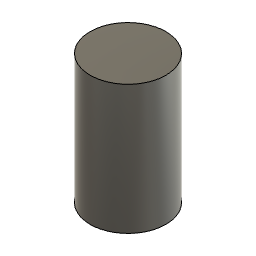
Busylight v2 (Autodesk Fusion 360 design; units mm, degrees)
Autodesk Fusion 360 part; units mm, degrees
sketch "Esquisse1" plane through (0, 0, 0) normal (0, 1, 0) x (1, 0, 0)
  circle A0 centre (0, 0) radius 12.5
  line L0 (12.5, 0) -> (0.5, 0) construction
  line L1 (-12.5, 0) -> (-4.5, 0) construction
  line L2 (-4.5, 6.25) -> (0.5, 6.25)
  line L3 (0.5, 6.25) -> (0.5, -6.25)
  line L4 (0.5, -6.25) -> (-4.5, -6.25)
  line L5 (-4.5, -6.25) -> (-4.5, 6.25)
  dimension "d1" = 25
  dimension "d2" = 12
  dimension "d3" = 8
  dimension "d4" = 12.5
  constraint coincident A0.centre origin
  constraint coincident A0 L0.start
  constraint horizontal L0
  constraint horizontal L1
  constraint coincident A0 L1.start
  constraint horizontal L2
  constraint vertical L3
  constraint horizontal L4
  constraint vertical L5
  constraint midpoint L0.end L3
  measures "d1" diameter of A0
  measures "d2" distance of L0.start L0.end
  measures "d3" distance of L1.start L1.end
  measures "d4" distance of L2.start L4.end
extrude "Extrusion1" add sketch "Esquisse1" along normal blind 2 makes body 1
sketch "Esquisse2" plane through (0, 2, 0) normal (0, 1, 0) x (-1, 0, 0)
  line L0 (-0.5, 6.25) -> (4.5, 6.25)
  line L1 (4.5, 6.25) -> (4.5, -6.25)
  line L2 (4.5, -6.25) -> (-0.5, -6.25)
  line L3 (-0.5, -6.25) -> (-0.5, 6.25)
  circle A0 centre (0, 0) radius 12.5
  line L4 (4.5, -6.25) -> (-0.5, 6.25) construction
  line L5 (-0.5, -6.25) -> (4.5, 6.25) construction
  line L6 (-1.5, 7.5) -> (5.5, 7.5)
  line L7 (5.5, 7.5) -> (5.5, -7.5)
  line L8 (5.5, -7.5) -> (-1.5, -7.5)
  line L9 (-1.5, -7.5) -> (-1.5, 7.5)
  line L10 (-1.5, 7.5) -> (5.5, -7.5) construction
  line L11 (5.5, 7.5) -> (-1.5, -7.5) construction
  line L12 (-3.5, 9.5) -> (7.5, 9.5)
  line L13 (7.5, 9.5) -> (7.5, -9.5)
  line L14 (7.5, -9.5) -> (-3.5, -9.5)
  line L15 (-3.5, -9.5) -> (-3.5, 9.5)
  point P0 (2, 0)
  dimension "d7" = 7
  dimension "d8" = 15
  dimension "d9" = -2
  constraint coincident L1.end L2.start
  constraint coincident L0.start L3.end
  constraint coincident L2.end L3.start
  constraint coincident L0.end L1.start
  constraint horizontal L6
  constraint perpendicular L6 L7
  constraint parallel L6 L8
  constraint parallel L7 L9
  constraint coincident L10 P0
  constraint coincident L11 P0
  constraint midpoint L4 P0
  measures "d7" distance of L7.end L8.end
  measures "d8" distance of L6.end L7.end
extrude "Extrusion2" add sketch "Esquisse2" along normal blind 5 contours L12 L13 L14 L15 bodies 1
sketch "Esquisse3" plane through (0, 7, 0) normal (0, 1, 0) x (-1, 0, 0)
  line L0 (5.5, -7.5) -> (-1.5, -7.5)
  line L1 (-1.5, -7.5) -> (-1.5, 7.5)
  line L2 (-1.5, 7.5) -> (5.5, 7.5)
  line L3 (5.5, 7.5) -> (5.5, -7.5)
  line L4 (-3.5, -9.5) -> (7.5, -9.5)
  line L5 (7.5, -9.5) -> (7.5, 9.5)
  line L6 (7.5, 9.5) -> (-3.5, 9.5)
  line L7 (-3.5, 9.5) -> (-3.5, -9.5)
  line L8 (5.5, -7.5) -> (-1.5, -7.5)
  line L9 (-1.5, -7.5) -> (-1.5, -9.5)
  line L10 (-1.5, -9.5) -> (5.5, -9.5)
  line L11 (5.5, -9.5) -> (5.5, -7.5)
  line L12 (5.5, 7.5) -> (-1.5, 7.5)
  line L13 (-1.5, 7.5) -> (-1.5, 9.5)
  line L14 (-1.5, 9.5) -> (5.5, 9.5)
  line L15 (5.5, 9.5) -> (5.5, 7.5)
  constraint horizontal L8
  constraint vertical L9
  constraint horizontal L10
  constraint vertical L11
  constraint coincident L4 L9.end
  constraint coincident L0.start L3.end
  constraint horizontal L12
  constraint vertical L13
  constraint horizontal L14
  constraint vertical L15
  constraint coincident L6 L13.end
  constraint coincident L2.end L3.start
extrude "Extrusion3" add sketch "Esquisse3" along normal blind 5.5 contours L0 L4 L8 L9 L10 L11 | L2 L6 L12 L13 L14 L15 bodies 1
sketch "Esquisse4" plane through (0, 12.5, 0) normal (0, 1, 0) x (-1, 0, 0)
  line L0 (5.5, -9.5) -> (5.5, -7.5)
  line L1 (5.5, -7.5) -> (-1.5, -7.5)
  line L2 (-1.5, -7.5) -> (-1.5, -9.5)
  line L3 (-1.5, -9.5) -> (5.5, -9.5)
  line L4 (5.5, 7.5) -> (-1.5, 7.5)
  line L5 (-1.5, 7.5) -> (-1.5, 5.5)
  line L6 (-1.5, 5.5) -> (5.5, 5.5)
  line L7 (5.5, 5.5) -> (5.5, 7.5)
  line L8 (5.5, -7.5) -> (-1.5, -7.5)
  line L9 (-1.5, -7.5) -> (-1.5, -5.5)
  line L10 (-1.5, -5.5) -> (5.5, -5.5)
  line L11 (5.5, -5.5) -> (5.5, -7.5)
  constraint horizontal L4
  constraint vertical L5
  constraint horizontal L6
  constraint vertical L7
  constraint horizontal L8
  constraint vertical L9
  constraint horizontal L10
  constraint vertical L11
  constraint coincident L0.end L1.start
extrude "Extrusion4" add sketch "Esquisse4" 1 faces at (-0.8333, 12.5, 8.8333) along normal blind 2 on bodies 1 bodies 1
sketch "Esquisse5" plane through (0, 0, 9.5) normal (0, 0, 1) x (1, 0, 0)
  line L0 (-7.5, 2) -> (3.5, 2)
  line L1 (3.5, 2) -> (3.5, 7)
  line L2 (3.5, 7) -> (1.5, 7)
  line L3 (1.5, 7) -> (1.5, 14.5)
  line L4 (1.5, 14.5) -> (-5.5, 14.5)
  line L5 (-5.5, 14.5) -> (-5.5, 7)
  line L6 (-5.5, 7) -> (-7.5, 7)
  line L7 (-7.5, 7) -> (-7.5, 2)
  line L8 (-5.5, 7) -> (-5.5, 2)
  line L9 (-6.5, 7) -> (-6.5, 2)
  line L10 (1.5, 7) -> (1.5, 2)
  line L11 (2.5, 7) -> (2.5, 2)
  dimension "d18" = 1
  dimension "d19" = -1
  constraint coincident L5.end L6.start
  constraint coincident L0 L8.end
  constraint perpendicular L0 L8
  constraint coincident L2.end L3.start
  constraint coincident L0 L10.end
  constraint perpendicular L0 L10
sketch "Esquisse6" plane through (0, 0, -9.5) normal (0, 0, -1) x (-1, 0, 0)
  line L0 (-3.5, 2) -> (7.5, 2)
  line L1 (7.5, 2) -> (7.5, 7)
  line L2 (7.5, 7) -> (5.5, 7)
  line L3 (5.5, 7) -> (5.5, 14.5)
  line L4 (5.5, 14.5) -> (-1.5, 14.5)
  line L5 (-1.5, 14.5) -> (-1.5, 7)
  line L6 (-1.5, 7) -> (-3.5, 7)
  line L7 (-3.5, 7) -> (-3.5, 2)
  line L8 (-1.5, 7) -> (-1.5, 2)
  line L9 (5.5, 7) -> (5.5, 2)
  line L10 (-2.5, 7) -> (-2.5, 2)
  line L11 (6.5, 7) -> (6.5, 2)
  dimension "d20" = 1
  dimension "d21" = -1
  constraint coincident L5.end L6.start
  constraint coincident L0 L8.end
  constraint perpendicular L0 L8
  constraint coincident L2.end L3.start
  constraint coincident L0 L9.end
  constraint perpendicular L0 L9
extrude "Extrusion7" add 1 faces at (6.5, 2, 0) along direction (0, 1, 0) blind 2 separate body on bodies 1 makes body 2
ref_plane "Plan de construction1" through (0, 2, 0) normal (0, 1, 0) x (1, 0, 0)
split "Scinder1" by plane through (0, 2, 0) normal (0, 1, 0) bodies 1 makes body 3 at (-0.8333, 9.5, 9.5)
move_body "Déplacer1" bodies 3 to x (1, 0, 0) y (0, 1, 0) z (0, 0, 1) at (0, 10, 0)
combine "Combiner1" operation add target body 2 tool bodies 1
sketch "Esquisse7" plane through (0, 4, 0) normal (0, 1, 0) x (-1, 0, 0)
  circle A0 centre (0, 0) radius 12.5
  line L0 (-3.5, -9.5) -> (-3.5, 9.5)
  line L1 (-3.5, 9.5) -> (7.5, 9.5)
  line L2 (7.5, 9.5) -> (7.5, -9.5)
  line L3 (7.5, -9.5) -> (-3.5, -9.5)
  circle A1 centre (0, 0) radius 16.5
  circle A2 centre (0, 0) radius 18.5
  dimension "d33" = 33
  dimension "d34" = 2
  constraint coincident A0.centre A1.centre
  measures "d33" diameter of A1
extrude "Extrusion8" add sketch "Esquisse7" against normal blind 2 contours A0 | A1 | A2 bodies 2
extrude "Extrusion9" add sketch "Esquisse7" against normal blind 15 contours A2 bodies 2
extrude "Extrusion10" add 1 faces at (-0.8333, 19.5, 9.5) along direction (0, 0, 1) blind 2 on bodies 3 bodies 3
extrude "Extrusion11" add 2 faces at (-3.1667, 13.6667, -9.5) (-0.8333, 23.1667, -9.5) along direction (0, 0, -1) blind 2 on bodies 3 bodies 3
extrude "Extrusion12" cut 1 faces at (-0.1667, 2.6667, 9.5) along direction (0, 0, 1) blind 2.25 on bodies 2 bodies 2
extrude "Extrusion13" cut 1 faces at (-3.8333, 2.6667, -9.5) along direction (0, 0, -1) blind 2.25 on bodies 2 bodies 2
extrude "Extrusion14" cut 1 faces at (-7.5, 3.3333, 3.3333) along direction (-1, 0, 0) blind 0.25 on bodies 2 bodies 2
extrude "Extrusion15" cut 1 faces at (3.5, 2.6667, 3.9167) along direction (1, 0, 0) blind 0.25 on bodies 2 bodies 2
extrude "Extrusion16" add 2 faces at (-0.8333, 24.5, -7.5) (-3.1667, 24.5, 9.5) along direction (0, 1, 0) blind 1 on bodies 3 bodies 3
sketch "Esquisse8" plane through (0, 4, 0) normal (0, 1, 0) x (-1, 0, 0)
  circle A0 centre (0, 0) radius 18.5
  line L0 (7.75, -11.75) -> (-3.75, -11.75)
  line L1 (-3.75, -11.75) -> (-3.75, 11.75)
  line L2 (-3.75, 11.75) -> (7.75, 11.75)
  line L3 (7.75, 11.75) -> (7.75, -11.75)
  circle A1 centre (0, 0) radius 20
  line L4 (7.75, -11.75) -> (-3.75, -11.75)
  line L5 (-3.75, -11.75) -> (-3.75, 11.75)
  line L6 (-3.75, 11.75) -> (7.75, 11.75)
  line L7 (7.75, 11.75) -> (7.75, -11.75)
  line L8 (17.5, 0) -> (-17.5, 0) construction
  line L9 (0, -17.5) -> (0, 17.5) construction
  circle A2 centre (0, -17.5) radius 1.5
  circle A3 centre (17.5, 0) radius 1.5
  circle A4 centre (-17.5, 0) radius 1.5
  circle A5 centre (0, 17.5) radius 1.5
  circle A6 centre (0, -17.5) radius 0.75
  circle A7 centre (0, 17.5) radius 0.75
  circle A8 centre (0, 0) radius 17.5 construction
  line L10 (0, 0) -> (-14.3352, -10.0376) construction
  line L11 (0, 0) -> (17.5, 0) construction
  circle A9 centre (-14.3352, -10.0376) radius 1.5
  dimension "d53" = 40
  dimension "d61" = 35
  dimension "d64" = 35
  dimension "d65" = 3
  dimension "d66" = 3
  dimension "d67" = 3
  dimension "d68" = 3
  dimension "d73" = 1.5
  dimension "d74" = 1.5
  dimension "d79" = 145
  dimension "d80" = 3
  constraint coincident A0.centre A1.centre
  constraint horizontal L4
  constraint vertical L5
  constraint horizontal L6
  constraint vertical L7
  constraint coincident L1.end L2.start
  constraint coincident L0.start L3.end
  constraint horizontal L8
  constraint midpoint A0.centre L8
  constraint vertical L9
  constraint midpoint A0.centre L9
  constraint coincident L9.start A2.centre
  constraint coincident L9.end A5.centre
  constraint concentric A2 A6
  constraint concentric A5 A7
  constraint concentric A1 A8
  constraint coincident L8.end A8
  constraint horizontal L11
  constraint coincident L10.end A9.centre
  measures "d53" diameter of A1
  measures "d61" distance of L8.start L8.end
  measures "d64" distance of L9.start L9.end
  measures "d65" diameter of A2
  measures "d66" diameter of A3
  measures "d67" diameter of A4
  measures "d68" diameter of A5
  measures "d73" diameter of A6
  measures "d74" diameter of A7
  measures "d79" angle of L10 L11
  measures "d80" diameter of A9
extrude "Extrusion19" add sketch "Esquisse8" along normal blind 2 separate body contours A0 A3 | A0 A3 | A0 A2 A3 A4 A5 A9 | A0 A5 | A0 A5 | A0 A2 | A0 A2 | A0 A4 | A0 A4 | A0 A9 | A0 A9 | A1 | A6 | A7 makes body 4
extrude "Extrusion20" add sketch "Esquisse8" along normal blind 4 contours A0 A3 | A0 A3 | A0 A5 | A0 A5 | A0 A2 | A0 A2 | A0 A4 | A0 A4 | A6 | A7 bodies 4
extrude "Extrusion22" add sketch "Esquisse8" along normal blind 6 contours A6 | A7 bodies 4
extrude "Extrusion23" cut 1 faces at (17.0869, 8, 0.2817) along direction (0, -1, 0) blind 2 on bodies 4 bodies 4
extrude "Extrusion24" add sketch "Esquisse8" along normal blind 4 contours A0 A9 | A0 A9 bodies 4
sketch "Esquisse10" plane through (0, 6, 0) normal (0, 1, 0) x (-1, 0, 0)
  circle A0 centre (-14.3352, -10.0376) radius 1.5
  circle A1 centre (0, -17.5) radius 1.5
  circle A2 centre (17.5, 0) radius 1.5
  circle A3 centre (0, 17.5) radius 1.5
  line L0 (-3.75, 11.75) -> (7.75, 11.75)
  line L1 (7.75, 11.75) -> (7.75, -11.75)
  line L2 (7.75, -11.75) -> (-3.75, -11.75)
  line L3 (-3.75, -11.75) -> (-3.75, 11.75)
  circle A4 centre (0, 0) radius 20
  circle A5 centre (0, 0) radius 12.5 construction
  line L4 (12, 2.5) -> (9, 2.5)
  line L5 (9, 2.5) -> (9, -2.5)
  line L6 (9, -2.5) -> (12, -2.5)
  line L7 (12, -2.5) -> (12, 2.5)
  line L8 (7.75, 0) -> (12.5, 0) construction
  line L9 (12, 2.5) -> (9, -2.5) construction
  line L10 (9, 2.5) -> (12, -2.5) construction
  line L11 (-6.625, 2.5) -> (-9.625, 2.5)
  line L12 (-9.625, 2.5) -> (-9.625, -2.5)
  line L13 (-9.625, -2.5) -> (-6.625, -2.5)
  line L14 (-6.625, -2.5) -> (-6.625, 2.5)
  line L15 (-6.625, 2.5) -> (-9.625, -2.5) construction
  line L16 (-6.625, -2.5) -> (-9.625, 2.5) construction
  line L17 (7.75, 3.75) -> (7.75, -3.75)
  line L18 (7.75, -3.75) -> (13.25, -3.75)
  line L19 (13.25, -3.75) -> (13.25, 3.75)
  line L20 (13.25, 3.75) -> (7.75, 3.75)
  line L21 (-3.75, 0) -> (-12.5, 0) construction
  line L22 (-11.625, 4.5) -> (-11.625, -4.5)
  line L23 (-11.625, -4.5) -> (-4.625, -4.5)
  line L24 (-4.625, -4.5) -> (-4.625, 4.5)
  line L25 (-4.625, 4.5) -> (-11.625, 4.5)
  point P0 (10.5, 0)
  point P1 (-8.125, 0)
  dimension "d83" = 25
  dimension "d84" = 3
  dimension "d85" = 5
  dimension "d86" = 3
  dimension "d87" = 5
  dimension "d88" = 1.25
  dimension "d89" = 2
  constraint concentric A4 A5
  constraint horizontal L4
  constraint vertical L5
  constraint horizontal L6
  constraint vertical L7
  constraint midpoint L1 L8.start
  constraint coincident A5 L8.end
  constraint perpendicular L1 L8
  constraint horizontal L11
  constraint vertical L12
  constraint horizontal L13
  constraint vertical L14
  constraint midpoint L9 P0
  constraint coincident L8 P0
  constraint coincident L8.start L17
  constraint midpoint L3 L21.start
  constraint coincident A5 L21.end
  constraint perpendicular L3 L21
  constraint midpoint L16 P1
  constraint coincident L21 P1
  constraint midpoint L21 P1
  measures "d83" diameter of A5
  measures "d84" distance of L4.start L4.end
  measures "d85" distance of L4.start L6.end
  measures "d86" distance of L11.start L11.end
  measures "d87" distance of L11.start L13.end
extrude "Extrusion25" add sketch "Esquisse10" along normal blind 2 contours L1 L17 L18 L19 L20 | L22 L23 L24 L25 bodies 4
extrude "Extrusion26" add sketch "Esquisse10" along normal blind 55 separate body contours L4 L5 L6 L7 | L11 L12 L13 L14 makes body 5 at (-12, 24.3333, -0.8333) makes body 6 at (6.625, 24.3333, -0.8333)
copy_body "Copier/Coller des corps1" bodies 4 makes body 7
move_body "Déplacer3" bodies 7 to x (1, 0, 0) y (0, -1, 0) z (0, 0, -1) at (0, 67, 0)
sketch "Esquisse11" plane through (0, 63, 0) normal (0, 1, 0) x (-1, 0, 0)
  line L0 (7.75, -11.75) -> (-3.75, -11.75)
  line L1 (-3.75, -11.75) -> (-3.75, 11.75)
  line L2 (-3.75, 11.75) -> (7.75, 11.75)
  line L3 (7.75, 11.75) -> (7.75, -11.75)
  circle A0 centre (0, 0) radius 20
  line L4 (7.75, -11.75) -> (-3.75, -11.75)
  line L5 (-3.75, -11.75) -> (-3.75, 11.75)
  line L6 (-3.75, 11.75) -> (7.75, 11.75)
  line L7 (7.75, 11.75) -> (7.75, -11.75)
  constraint horizontal L4
  constraint vertical L5
  constraint horizontal L6
  constraint vertical L7
  constraint coincident L1.end L2.start
  constraint coincident L0.start L3.end
extrude "Extrusion27" add sketch "Esquisse11" against normal blind 2 contours L0 L1 L2 L3 L4 L5 L6 L7 bodies 7
sketch "Esquisse13" plane through (0, 63, 0) normal (0, 1, 0) x (-1, 0, 0)
  circle A0 centre (0, 0) radius 20
  circle A1 centre (0, 0) radius 20
  circle A2 centre (0, 0) radius 20.8
  dimension "d101" = 0.8
  constraint coincident A0.centre A1.centre
extrude "Extrusion30" add sketch "Esquisse13" against normal blind 60 separate body contours A0 A1 | A2 makes body 8
extrude "Extrusion31" add 1 faces at (-0.247, 63, -5.7261) along direction (0, 1, 0) blind 1 on bodies 8 bodies 8
ref_plane "Plan de construction2" through (0, -106, 0) normal (0, -1, 0) x (1, 0, 0)
sketch "Esquisse14" plane through (0, -106, 0) normal (0, -1, 0) x (-1, 0, 0)
  circle A0 centre (0, 0) radius 16.5
  circle A1 centre (0, 0) radius 18.5
  dimension "d108" = 33
  dimension "d109" = 2
  constraint coincident A0.centre A1.centre
  measures "d108" diameter of A0
extrude "Extrusion32" add sketch "Esquisse14" along normal blind 4 separate body contours A0 | A1 makes body 9
extrude "Extrusion33" add sketch "Esquisse14" against normal blind 50 bodies 9
sketch "Esquisse15" plane through (0, -110, 0) normal (0, -1, 0) x (1, 0, 0)
  circle A0 centre (0, 0) radius 18.5
  circle A1 centre (-10.3, 0) radius 6.2
  line L0 (0, 18.5) -> (0, -18.5) construction
  line L1 (-18.5, 0) -> (18.5, 0) construction
  circle A2 centre (0, 0) radius 16.5 construction
  circle A3 centre (10.3, 0) radius 6.2
  circle A4 centre (0, 10.3) radius 6.2
  circle A5 centre (0, -10.3) radius 6.2
  dimension "d114" = 12.4
  dimension "d115" = 12.4
  dimension "d116" = 12.4
  dimension "d117" = 12.4
  constraint coincident A0 L0.start
  constraint coincident A0 L0.end
  constraint vertical L0
  constraint coincident A0 L1.start
  constraint coincident A0 L1.end
  constraint perpendicular L0 L1
  constraint coincident A1.centre L1
  constraint tangent A1 A2
  constraint coincident L1 A3.centre
  constraint tangent A2 A3
  constraint coincident L0 A4.centre
  constraint coincident L0 A5.centre
  constraint tangent A2 A4
  constraint tangent A2 A5
  measures "d114" diameter of A1
  measures "d115" diameter of A3
  measures "d116" diameter of A4
  measures "d117" diameter of A5
extrude "Extrusion34" cut sketch "Esquisse15" against normal blind 2.4 contours A1 | A3 | A4 | A5 bodies 9
extrude "Extrusion35" cut 1 faces at (9.625, 6.6667, 0.8333) along direction (1, 0, 0) blind 0.2 on bodies 4 bodies 4
extrude "Extrusion36" cut 1 faces at (7.6917, 6.6667, 2.5) along direction (0, 0, 1) blind 0.2 on bodies 4 bodies 4
extrude "Extrusion37" cut 1 faces at (-11, 6.6667, 2.5) along direction (0, 0, 1) blind 0.2 on bodies 4 bodies 4
extrude "Extrusion38" cut 1 faces at (-12, 6.6667, -0.7667) along direction (-1, 0, 0) blind 0.2 on bodies 4 bodies 4
extrude "Extrusion39" cut 1 faces at (7.625, 59.6667, 2.5) along direction (0, 0, 1) blind 0.2 on bodies 7 bodies 7
extrude "Extrusion40" cut 1 faces at (9.625, 60.3333, -0.7667) along direction (1, 0, 0) blind 0.2 on bodies 7 bodies 7
extrude "Extrusion41" cut 1 faces at (-10, 60.3333, 2.5) along direction (0, 0, 1) blind 0.2 on bodies 7 bodies 7
extrude "Extrusion42" cut 1 faces at (-12, 59.6667, 0.9667) along direction (-1, 0, 0) blind 0.2 on bodies 7 bodies 7
extrude "Extrusion43" add 2 faces at (-11, 6, -0.8333) (8.625, 6, 0.8333) along direction (0, -1, 0) blind 10 on bodies 5 6 bodies 5 6
extrude "Extrusion44" add 1 faces at (-0.247, 3, -5.7261) along direction (0, -1, 0) blind 10 on bodies 8 bodies 8
hidden bodies 3 2 4 5 6 7 9
named bodies: "proto 1", "USB plate", "USB holder", "LED support bottom", "Raiser #1", "Raiser #2", "LED base bottom", "LED support top", "LED cover", "BusyLight magnetic support"
